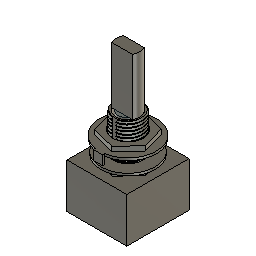
OVHD_External_Lights_Panel (Autodesk Fusion 360 archive; units mm, degrees)
design "Toggle_Switch_v2"
Autodesk Fusion 360 part; units mm, degrees
sketch "Sketch1" plane through (0, 0, 0) normal (0, 0, 1) x (1, 0, 0)
  line L0 (6.35, 6.6) -> (-6.35, 6.6)
  line L1 (-6.35, 6.6) -> (-6.35, -6.6)
  line L2 (-6.35, -6.6) -> (6.35, -6.6)
  line L3 (6.35, -6.6) -> (6.35, 6.6)
  line L4 (6.35, 6.6) -> (-6.35, -6.6) construction
  line L5 (-6.35, 6.6) -> (6.35, -6.6) construction
  dimension "d1" = 12.7
  dimension "d2" = 13.2
  constraint horizontal L0
  constraint perpendicular L0 L1
  constraint parallel L0 L2
  constraint parallel L1 L3
  constraint coincident L4 origin
  constraint coincident L5 origin
  measures "d1" distance of L1.end L2.end
  measures "d2" distance of L0.end L1.end
extrude "Extrude1" add sketch "Sketch1" against normal blind 9.5 makes body 1
sketch "Sketch2" plane through (0, 0, 0) normal (0, 0, 1) x (1, 0, 0)
  circle A0 centre (0, 0) radius 3
  dimension "d5" = 6
  constraint coincident A0.centre origin
  measures "d5" diameter of A0
extrude "Extrude2" add sketch "Sketch2" along normal blind 9 bodies 1
sketch "Sketch3" plane through (0, 0, 9) normal (0, 0, 1) x (-1, 0, 0)
  circle A0 centre (0, 0) radius 3
  line L0 (-0.5, 3.25) -> (0.5, 3.25)
  line L1 (0.5, 3.25) -> (0.5, 2.75)
  line L2 (0.5, 2.75) -> (-0.5, 2.75)
  line L3 (-0.5, 2.75) -> (-0.5, 3.25)
  line L4 (-0.5, 3.25) -> (0.5, 2.75) construction
  line L5 (0.5, 3.25) -> (-0.5, 2.75) construction
  point P0 (0, 3)
  dimension "d8" = 1
  dimension "d9" = 0.5
  constraint horizontal L0
  constraint perpendicular L0 L1
  constraint parallel L0 L2
  constraint parallel L1 L3
  constraint coincident L4 P0
  constraint coincident L5 P0
  constraint coincident A0 P0
  measures "d8" distance of L1.end L2.end
  measures "d9" distance of L0.end L1.end
shell "Shell1" thickness 0.5 removed faces 1 at (-1.1591, 0.5829, 9) on bodies 1
extrude "Extrude3" cut sketch "Sketch3" against normal blind 9 contours A0 L1 L2 L3 | A0 L0 L1 L3 picked at (-0.0558, 2.8318) bodies 1
thread "Thread1" "ANSI Unified Screw Threads 0.25 1/4-40 UNS 1/4-40 UNS 2A" major diameter 6.2636 minor diameter 5.5702 pitch 0.635 angle 60 modelled right hand crest width 0.0961 on face at (-0.646, -2.9296, 6) crest through (3.1318, 0, -0.1588) on bodies 1
sketch "Sketch4" plane through (0, 0, 0) normal (0, 0, 1) x (1, 0, 0)
  circle A0 centre (0, 0) radius 2
  dimension "d15" = 4
  constraint coincident A0.centre origin
  measures "d15" diameter of A0
extrude "Extrude4" add sketch "Sketch4" along normal blind 9 separate body makes body 2
sketch "Sketch5" plane through (0, 0, 9) normal (0, 0, 1) x (-1, 0, 0)
  circle A0 centre (0, 0) radius 2
  line L0 (2.1651, -1.25) -> (-2.1651, -1.25)
  line L1 (-2.1651, 1.25) -> (2.1651, 1.25)
  line L2 (-1.25, 2.5) -> (1.25, -2.5) construction
  line L3 (1.25, 2.5) -> (-1.25, -2.5) construction
  arc A1 (-2.1651, 1.25) -> (-2.1651, -1.25) centre (0, 0) ccw
  arc A2 (2.1651, -1.25) -> (2.1651, 1.25) centre (0, 0) ccw
  dimension "d18" = 5
  dimension "d19" = 2.5
  constraint coincident A0.centre A1.centre
  constraint parallel L0 L1
  constraint coincident L2 A0.centre
  constraint coincident L3 A0.centre
  constraint concentric A1 A2
  measures "d18" diameter of A1
  measures "d19" distance of L2.end L3.end
extrude "Extrude5" add sketch "Sketch5" along normal blind 12 contours A0 L0 L1 | A0 L0 L1 A2 | A0 L0 L1 A1 bodies 1 2
sketch "Sketch6" plane through (0, 0, 0) normal (0, 0, 1) x (-1, 0, 0)
  line L0 (-6.35, 6.6) -> (-6.35, -6.6)
  line L1 (-6.35, -6.6) -> (6.35, -6.6)
  line L2 (6.35, -6.6) -> (6.35, 6.6)
  line L3 (6.35, 6.6) -> (-6.35, 6.6)
  line L4 (-0.4408, 2.75) -> (0.4408, 2.75)
  arc A0 (1.7635, 2.1557) -> (0.4408, 2.75) centre (0, 0) ccw
  spline S0 degree 3 poles (1.7635, 2.1557) (1.9265, 2.0386) (2.0763, 1.9042) (2.3466, 1.604) (2.4659, 1.4386) (2.7529, 0.9352) (2.8728, 0.5749) (2.9704, -0.1801) (2.9439, -0.5679) (2.7431, -1.3206) (2.5674, -1.6773) (2.0851, -2.3114) (1.7804, -2.5807) (1.433, -2.7847) knots -0.589294 -0.589294 -0.589294 -0.589294 -0.528968 -0.528968 -0.467844 -0.467844 -0.35479 -0.35479 -0.23913 -0.23913 -0.120866 -0.120866 0 0 0 0
  arc A1 (-1.433, -2.7847) -> (1.433, -2.7847) centre (0, 0) ccw
  spline S1 degree 3 poles (-1.433, -2.7847) (-1.6253, -2.6718) (-1.805, -2.5386) (-2.1305, -2.2377) (-2.2758, -2.0713) (-2.627, -1.5684) (-2.7876, -1.2058) (-2.9574, -0.4475) (-2.9681, -0.06) (-2.8403, 0.6885) (-2.7063, 1.0428) (-2.3133, 1.6717) (-2.061, 1.942) (-1.7635, 2.1557) knots -0.587839 -0.587839 -0.587839 -0.587839 -0.521083 -0.521083 -0.455123 -0.455123 -0.337445 -0.337445 -0.222364 -0.222364 -0.109882 -0.109882 0 0 0 0
  arc A2 (-0.4408, 2.75) -> (-1.7635, 2.1557) centre (0, 0) ccw
  line L5 (-4.8507, 1.2127) -> (-3.4756, -3.5945)
  line L6 (-3.4756, -3.5945) -> (1.3751, -4.8072)
  line L7 (1.3751, -4.8072) -> (4.8507, -1.2127)
  line L8 (4.8507, -1.2127) -> (3.4756, 3.5945)
  line L9 (3.4756, 3.5945) -> (-1.3751, 4.8072)
  line L10 (-1.3751, 4.8072) -> (-4.8507, 1.2127)
  circle A3 centre (0, 0) radius 3.25
  dimension "d22" = 5
  dimension "d23" = 6.5
  constraint coincident A0.centre A1.centre
  constraint concentric A0 A3
  measures "d22" distance of L5.start A0.centre
  measures "d23" diameter of A3
extrude "Extrude6" add sketch "Sketch6" along normal blind 1 separate body contours L5 L6 L7 L8 L9 L10 makes body 3
sketch "Sketch7" plane through (0, 0, 1) normal (0, 0, 1) x (-1, 0, 0)
  circle A0 centre (0, 0) radius 3.25
  line L0 (-1.3751, 4.8072) -> (-4.8507, 1.2127)
  line L1 (-4.8507, 1.2127) -> (-3.4756, -3.5945)
  line L2 (-3.4756, -3.5945) -> (1.3751, -4.8072)
  line L3 (1.3751, -4.8072) -> (4.8507, -1.2127)
  line L4 (4.8507, -1.2127) -> (3.4756, 3.5945)
  line L5 (3.4756, 3.5945) -> (-1.3751, 4.8072)
  circle A1 centre (0, 0) radius 6
  line L6 (0.3137, 3.2348) -> (0.3137, 2.925)
  line L7 (0.3137, 2.925) -> (-0.3363, 2.925)
  line L8 (-0.3363, 2.925) -> (-0.3363, 3.2326)
  line L9 (-0.3363, 3.575) -> (0.3137, 2.925) construction
  line L10 (0.3137, 3.575) -> (-0.3363, 2.925) construction
  arc A2 (-0.0113, 3.25) -> (0.3137, 3.2348) centre (0, 0) ccw
  dimension "d26" = 12
  dimension "d27" = 0.65
  dimension "d28" = 0.65
  constraint coincident A0.centre A1.centre
  constraint concentric A1 A2
  constraint parallel L6 L8
  constraint coincident L9 A2.start
  constraint coincident L10 A2.start
  constraint coincident A0 A2.start
  constraint coincident A0 L8.end
  measures "d26" diameter of A1
  measures "d27" distance of L6.end L7.end
  measures "d28" distance of L10.start L6.end
extrude "Extrude7" add sketch "Sketch7" along normal blind 0.5 separate body contours L0 L1 L2 L3 L4 L5 | A1 makes body 4
sketch "Sketch8" plane through (0, 0, 1.5) normal (0, 0, 1) x (-1, 0, 0)
  circle A0 centre (0, 0) radius 3.25
  circle A1 centre (0, 0) radius 6
  line L0 (0.9967, 5.8797) -> (-1.0033, 5.8797)
  line L1 (-1.0033, 5.8797) -> (-1.0033, 6.3797)
  line L2 (-1.0033, 6.3797) -> (0.9967, 6.3797)
  line L3 (0.9967, 6.3797) -> (0.9967, 5.8797)
  point P0 (0, -6)
  dimension "d31" = 2
  dimension "d32" = 0.5
  constraint horizontal L0
  constraint perpendicular L0 L1
  constraint parallel L0 L2
  constraint parallel L1 L3
  constraint coincident A1 P0
  measures "d31" distance of L1.end L2.end
  measures "d32" distance of L0.end L1.end
extrude "Extrude8" add sketch "Sketch8" along normal blind 1.5 contours A1 L0 L1 L3 | A1 L1 L2 L3 picked at (-0.1149, 5.9166) bodies 4
extrude "Extrude9" add 1 faces at (-0.1083, -6.2501, 1.5) along direction (0, 0, -1) blind 0.5 on bodies 4 bodies 4
copy_body "CopyPasteBodies1" bodies 3 makes body 5
move_body "Move1" bodies 5 to x (1, 0, 0) y (0, 1, 0) z (0, 0, 1) at (0, 0, 1.4)
sketch "Sketch9" plane through (0, 0, 9) normal (0, 0, 1) x (-1, 0, 0)
  line L0 (-1.5612, 1.25) -> (1.5612, 1.25)
  arc A0 (1.5612, 1.25) -> (-1.5612, 1.25) centre (0, 0) ccw
move_body "Move2" bodies 4 to x (-1, 0, 0) y (0, 1, 0) z (0, 0, -1) at (0, 0, 3)
move_body "Move3" bodies 5 to x (1, 0, 0) y (0, 1, 0) z (0, 0, 1) at (0, 0, 0.5)
move_body "Move4" bodies 5 to x (1, 0, 0) y (0, 1, 0) z (0, 0, 1) at (0, 0, 0.1)
sketch "Sketch10" plane through (0, 0, 1) normal (0, 0, 1) x (-1, 0, 0)
  circle A0 centre (0, 0) radius 3.25
  line L0 (-1.3751, 4.8072) -> (-4.8507, 1.2127)
  line L1 (-4.8507, 1.2127) -> (-3.4756, -3.5945)
  line L2 (-3.4756, -3.5945) -> (1.3751, -4.8072)
  line L3 (1.3751, -4.8072) -> (4.8507, -1.2127)
  line L4 (4.8507, -1.2127) -> (3.4756, 3.5945)
  line L5 (3.4756, 3.5945) -> (-1.3751, 4.8072)
  circle A1 centre (0, 0) radius 3.25
  circle A2 centre (0, 0) radius 5.75
  dimension "d49" = 11.5
  constraint concentric A0 A1
  constraint coincident A0.centre A1.centre
  measures "d49" diameter of A2
extrude "Extrude10" add sketch "Sketch10" along normal blind 0.5 contours L0 L1 L2 L3 L4 L5 | A2 bodies 3
move_body "Move5" bodies 5 4 to x (1, 0, 0) y (0, 1, 0) z (0, 0, 1) at (0, 0, 1.5)
ref_plane "WorkPlane1" through (0, -1.625, 0) normal (0, 0, 1) x (-1, 0, 0)
move_body "Move6" bodies 4 5 to x (1, 0, 0) y (0, 1, 0) z (0, 0, 1) at (0, 0, 2)
move_body "Move7" bodies 4 5 to x (1, 0, 0) y (0, 1, 0) z (0, 0, 1) at (0, 0, -2)
move_body "Move8" bodies 4 5 to x (1, 0, 0) y (0, 1, 0) z (0, 0, 1) at (0, 0, 1)
